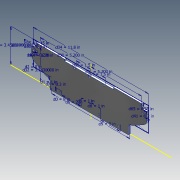
# Autodesk Inventor part: VP TRAY PUSHER PNL V2
Saved by Autodesk Inventor 2020.3 (Build 243373000, 373)
## iProperties
RuleStatus: InUse
AfterDocSave0: file://Part Number Cleaner
Created: 2019-10-29
Material: DELRIN 100, BLACK (EXTRUDED)
Vendor: HHMI: JRC - ID&F
Document SubType Name: Modeling
Designer: arnoldj
Density: 1.42 g/cm^3
Appearance: Aluminum - Flat
DESIGN DEPARTMENT: HHMI: JRC - ID&F
ALTERED ITEM PART NUMBER: N/A
ALTERED ITEM VENDOR: N/A
ALTERED ITEM DESCRIPTION: N/A
Author: arnoldj
Revision Number: 0
Autodesk Inventor part; units mm, degrees
ref_plane "YZ Plane" through (0, 0, 0) normal (1, 0, 0) x (0, 1, 0)
ref_plane "XZ Plane" through (0, 0, 0) normal (0, 1, 0) x (-1, 0, 0)
ref_plane "XY Plane" through (0, 0, 0) normal (0, 0, 1) x (1, 0, 0)
sketch "Sketch1" plane through (0, 0, 0) normal (0, 0, 1) x (1, 0, 0)
  line L0 (0, 105.156) -> (0, -17.526) projected
  line L1 (-209.804, 0) -> (209.804, 0) projected
  line L2 (101.6, 25.4) -> (-101.6, 25.4)
  line L3 (-101.6, 25.4) -> (-101.6, 0)
  line L4 (-101.6, 0) -> (101.6, 0)
  line L5 (101.6, 0) -> (101.6, 25.4)
  line L6 (101.6, 25.4) -> (-101.6, 0) construction
  line L7 (-101.6, 25.4) -> (101.6, 0) construction
  line L8 (149.86, 87.63) -> (-149.86, 87.63)
  line L9 (-149.86, 87.63) -> (-149.86, 25.4)
  line L10 (-149.86, 25.4) -> (149.86, 25.4)
  line L11 (149.86, 25.4) -> (149.86, 87.63)
  line L12 (149.86, 87.63) -> (-149.86, 25.4) construction
  line L13 (-149.86, 87.63) -> (149.86, 25.4) construction
  point P0 (0, 0)
  point P1 (0, 12.7)
  point P2 (0, 56.515)
  point P3 (-76.2, 7.62)
  point P4 (-25.4, 7.62)
  point P5 (25.4, 7.62)
  point P6 (76.2, 7.62)
  point P7 (-132.08, 79.8322)
  point P8 (132.08, 79.8322)
  point P9 (0, 79.8322)
  point P10 (-38.1, 79.8322)
  point P11 (38.1, 79.8322)
  dimension "d0" = 203.2
  dimension "d1" = 25.4
  dimension "d2" = 0
  dimension "d5" = 25.4
  dimension "d6" = 50.8
  dimension "d7" = 7.62
  dimension "d8" = 25.4
  dimension "d9" = 50.8
  dimension "d30" = 132.08
  dimension "d31" = 132.08
  dimension "d32" = 79.8322
  dimension "d33" = 87.63
  dimension "d34" = 299.72
  dimension "d62" = 38.1
  dimension "d63" = 38.1
  constraints: 24 end point, 5 horizontal alignment, 4 midpoint, 4 parallel, 4 point on line, 2 horizontal, 2 perpendicular
  measures "d0" distance of L3.end L4.end
  measures "d1" distance of L2.end L3.end
  measures "d2" distance between parallel lines of L10 L2
  measures "d5" distance from line of point (-25.4, 7.62) L0
  measures "d6" distance of point (-25.4, 7.62) point (-76.2, 7.62)
  measures "d7" distance from line of L4 point (-76.2, 7.62)
  measures "d8" distance from line of L0 point (25.4, 7.62)
  measures "d9" distance of point (25.4, 7.62) point (76.2, 7.62)
  measures "d30" distance from line of L0 point (-132.08, 79.832)
  measures "d31" distance from line of L0 point (132.08, 79.832)
  measures "d32" distance from line of L1 point (-132.08, 79.832)
  measures "d33" distance between parallel lines of L1 L8
  measures "d34" distance of L8.start L8.end
  measures "d62" distance from line of L0 point (-38.1, 79.832)
  measures "d63" distance from line of L0 point (38.1, 79.832)
extrude "Extrusion1" add sketch "Sketch1" along normal blind 4.4958
hole "Hole1" at (-76.2, 7.62, 0) at (-25.4, 7.62, 0) at (25.4, 7.62, 0) at (76.2, 7.62, 0) direction (0, 0, 1) diameter 3.1242 end through all
hole "Hole2" at (-132.08, 79.8322, 0) at (132.08, 79.8322, 0) at (0, 79.8322, 0) at (-38.1, 79.8322, 0) at (38.1, 79.8322, 0) direction (0, 0, 1) diameter 3.81 end through all clearance for "Socket Head Cap Screw" size "#6" standard "Ansi Unified Screw Threads"
sketch "Sketch2" plane through (0, 0, 0) normal (0, 0, 1) x (1, 0, 0)
  circle A0 centre (132.08, 79.8322) radius 1.905 projected
  circle A1 centre (-132.08, 79.8322) radius 1.905 projected
  circle A2 centre (0, 79.8322) radius 1.905 projected
  circle A3 centre (25.4, 7.62) radius 1.5621 projected
  circle A4 centre (-76.2, 7.62) radius 1.5621 projected
  circle A5 centre (-25.4, 7.62) radius 1.5621 projected
  circle A6 centre (76.2, 7.62) radius 1.5621 projected
  line L0 (-101.6, 25.4) -> (-101.6, 0) projected
  line L1 (-101.6, 0) -> (101.6, 0) projected
  line L2 (101.6, 0) -> (101.6, 25.4) projected
  line L3 (101.6, 25.4) -> (149.86, 25.4) projected
  line L4 (149.86, 25.4) -> (149.86, 87.63) projected
  line L5 (149.86, 87.63) -> (-149.86, 87.63) projected
  line L6 (-149.86, 87.63) -> (-149.86, 25.4) projected
  line L7 (-149.86, 25.4) -> (-101.6, 25.4) projected
  line L8 (-149.86, 87.63) -> (-137.16, 87.63)
  line L9 (-137.16, 87.63) -> (-137.16, 76.2)
  line L10 (-137.16, 76.2) -> (-149.86, 76.2)
  line L11 (-149.86, 76.2) -> (-149.86, 87.63)
  line L12 (149.86, 87.63) -> (137.16, 87.63)
  line L13 (137.16, 87.63) -> (137.16, 76.2)
  line L14 (137.16, 76.2) -> (149.86, 76.2)
  line L15 (149.86, 76.2) -> (149.86, 87.63)
  line L16 (-149.86, 87.63) -> (-149.2523, 87.63)
  line L17 (-149.2523, 87.63) -> (-151.5626, 87.63)
  line L18 (-151.5626, 87.63) -> (-149.86, 87.63)
  point P0 (0, 0)
  point P1 (-144.78, 67.945)
  point P2 (144.78, 67.945)
  point P3 (-138.43, 67.945)
  point P4 (138.43, 67.945)
  dimension "d35" = 11.43
  dimension "d36" = 12.7
  dimension "d39" = 8.255
  dimension "d40" = 5.08
  dimension "d41" = 5.08
  dimension "d64" = 6.35
  dimension "d65" = 6.35
  constraints: 22 end point, 4 parallel, 3 horizontal, 3 horizontal alignment, 2 equal length, 2 perpendicular, 1 collinear, 1 point on line
  measures "d35" distance of L8.end L9.end
  measures "d36" distance of L9.end L10.end
  measures "d39" distance from line of point (-144.78, 67.945) L10
  measures "d40" distance from line of point (-144.78, 67.945) L6
  measures "d41" distance from line of L4 point (144.78, 67.945)
  measures "d64" distance of point (-138.43, 67.945) point (-144.78, 67.945)
  measures "d65" distance of point (144.78, 67.945) point (138.43, 67.945)
extrude "Extrusion2" cut sketch "Sketch2" along normal up to next contours L6 L5 L9 L10 | L14 L13 L5 L4
hole "Hole3" at (-144.78, 67.945, 0) at (144.78, 67.945, 0) at (-138.43, 67.945, 0) at (138.43, 67.945, 0) direction (0, 0, 1) diameter 3.81 end through all clearance for "Socket Head Cap Screw" size "#6" standard "Ansi Unified Screw Threads"
sketch "Sketch3" plane through (0, 0, 0) normal (0, 0, 1) x (1, 0, 0)
  line L0 (0, 105.156) -> (0, -17.526) projected
  line L1 (-209.804, 0) -> (209.804, 0) projected
  line L2 (137.16, 87.63) -> (-137.16, 87.63) projected
  line L3 (63.5, 83.058) -> (-63.5, 83.058)
  line L4 (-63.5, 83.058) -> (-63.5, 87.63)
  line L5 (-63.5, 87.63) -> (63.5, 87.63)
  line L6 (63.5, 87.63) -> (63.5, 83.058)
  line L7 (63.5, 83.058) -> (-63.5, 87.63) construction
  line L8 (-63.5, 83.058) -> (63.5, 87.63) construction
  point P0 (0, 0)
  point P1 (0, 85.344)
  dimension "d49" = 4.572
  dimension "d50" = 127
  constraints: 12 end point, 2 midpoint, 2 parallel, 2 point on line, 1 horizontal, 1 perpendicular
  measures "d49" distance of L3.end L4.end
  measures "d50" distance of L3.start L3.end
extrude "Extrusion3" cut sketch "Sketch3" along normal up to next
fillet "Fillet1" radius 6.35 2 edges at (-137.16, 76.2, 2.2479) (137.16, 76.2, 2.2479)
chamfer "Chamfer1" distance 38.1 angle 30 1 edges at (149.86, 25.4, 2.2479) measured on face at (117.6867, 25.4, 1.4986)
chamfer "Chamfer2" distance 38.1 angle 30 1 edges at (-149.86, 25.4, 2.2479) measured on face at (-133.7733, 25.4, 1.4986)
fillet "Fillet2" radius 12.7 4 edges at (-149.86, 47.397, 2.2479) (-111.76, 25.4, 2.2479) (111.76, 25.4, 2.2479) (149.86, 47.397, 2.2479)
fillet "Fillet3" radius 6.35 2 edges at (-101.6, 25.4, 2.2479) (101.6, 25.4, 2.2479)
body "Solid1"
